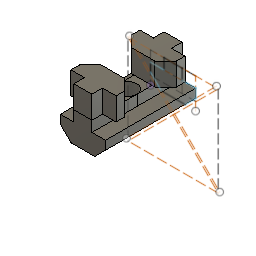
4040-t-conector v3 (Autodesk Fusion 360 design; units mm, degrees)
Autodesk Fusion 360 part; units mm, degrees
sketch "Sketch1" plane through (0, 0, 0) normal (0, 0, 1) x (1, 0, 0)
  line L0 (20, 0) -> (20, 13.5) construction
  line L1 (20, 13.5) -> (0, 13.5) construction
  line L2 (0, 13.5) -> (0, 0) construction
  line L3 (6, 13.5) -> (14, 13.5)
  line L4 (14, 13.5339) -> (14, 3.75) construction
  line L5 (14, 8.8) -> (6, 8.8) construction
  line L6 (6, 8.8) -> (6, 13.5) construction
  line L7 (0, 3.75) -> (20, 3.75) construction
  line L8 (-10, 13.5339) -> (30, 13.5339) construction
  line L9 (30, 13.5339) -> (30, -26.4661) construction
  line L10 (30, -26.4661) -> (-10, -26.4661) construction
  line L11 (-10, -26.4661) -> (-10, 13.5339) construction
  line L12 (-10, 13.5339) -> (30, -26.4661) construction
  line L13 (-9.2929, 14.241) -> (30.7071, -25.759) construction
  line L14 (30, 13.5339) -> (-10, -26.4661) construction
  line L15 (29.2929, 14.241) -> (-10.7071, -25.759) construction
  line L16 (0, 8.8) -> (20, 8.8) construction
  line L17 (6, 13.5) -> (6, 8.8)
  line L18 (0, 8.8) -> (0, 4.9481)
  line L19 (4.7481, 0.2) -> (15.2519, 0.2)
  line L20 (15.2519, 0.2) -> (20, 4.9481)
  line L21 (20, 4.9481) -> (20, 8.8)
  line L22 (20, 8.8) -> (14, 8.8)
  line L23 (14, 8.8) -> (14, 13.5)
  line L24 (6, 8.8) -> (0, 8.8)
  line L25 (0, 4.9481) -> (4.7481, 0.2)
  dimension "d1" = 20
  dimension "d2" = 13.5
  dimension "d3" = 8
  dimension "d4" = 4.7
  dimension "d5" = 6
  dimension "d6" = 9.75
  dimension "d7" = 40
  dimension "d8" = 40
  dimension "d9" = 10
  dimension "d10" = -1
  dimension "d11" = 1
  dimension "d21" = 13.3
  constraint vertical L0
  constraint horizontal L1
  constraint vertical L2
  constraint coincident L2.end origin
  constraint horizontal L3
  constraint vertical L4
  constraint horizontal L5
  constraint vertical L6
  constraint coincident L1 L3.start
  constraint coincident L2 L7.start
  constraint coincident L0 L7.end
  constraint perpendicular L0 L7
  constraint horizontal L8
  constraint vertical L9
  constraint horizontal L10
  constraint vertical L11
  constraint coincident L2 L16.start
  constraint coincident L0 L16.end
  constraint perpendicular L0 L16
  constraint coincident L13 L18.end
  constraint coincident L2 L18.end
  constraint coincident L13 L19.start
  constraint coincident L15 L19.end
  constraint coincident L15 L20.end
  constraint coincident L0 L20.end
  constraint coincident L7 L4.end
  constraint coincident L5.start L4
  constraint coincident L8 L4.start
  constraint coincident L3.end L4
  measures "d1" distance of L2.end L0.start
  measures "d2" distance of L2.end L1.end
  measures "d3" distance of L3.start L3.end
  measures "d4" distance of L3.start L5.end
  measures "d5" distance of L2 L6
  measures "d6" distance of L1 L7
  measures "d7" distance of L8.start L8.end
  measures "d8" distance of L8.start L10.end
  measures "d9" distance of L2 L11
  measures "d21" distance of L1 L19
extrude "Extrude1" add sketch "Sketch1" along normal blind 40 makes body 1
sketch "Sketch3" plane through (0, 0, 0) normal (0, 0, 1) x (1, 0, 0)
copy_body "CopyPasteBodies2" bodies 1 makes body 2
copy_body "CopyPasteBodies3" bodies 1 makes body 3
move_body "Move3" bodies 3 to x (1, 0, 0) y (0, 0, 1) z (0, -1, 0) at (0, 53.5, 26.5)
copy_body "CopyPasteBodies4" bodies 1 makes body 4
move_body "Move4" bodies 4 to x (1, 0, 0) y (0, 0, -1) z (0, 1, 0) at (0, 13.5, 13.5)
move_face "OffsetFaces1" offset -30 1 faces at (8.6667, 53.5, 29.5667) on bodies 3
move_face "OffsetFaces2" offset -20 1 faces at (8.6667, 53.5, 10.4333) on bodies 4
sketch "Sketch4" plane through (0, 13.5, 0) normal (0, 1, 0) x (-1, 0, 0)
  line L0 (-14, 0) -> (-6, 0)
  line L1 (-6, 0) -> (-6, 40)
  line L2 (-6, 40) -> (-14, 40)
  line L3 (-14, 40) -> (-14, 0)
  circle A0 centre (-10, 20) radius 4
  line L4 (0, 0) -> (0, 40)
  line L5 (-20, 0) -> (-20, 40)
  dimension "d16" = 8
  dimension "d17" = 20
  dimension "d18" = 10
  dimension "d22" = 20
  measures "d16" diameter of A0
  measures "d17" distance of L0 A0.centre
  measures "d18" distance of A0.centre L4
  measures "d22" distance of L4 L5
extrude "Extrude2" cut sketch "Sketch4" against normal blind 17 contours A0 bodies 1 2
combine "Combine1" operation add target body 3 tool bodies 1 4
copy_body "Body->Comp1" bodies 2 removing the originals makes body 5 in component "t-block"
move_face "OffsetFaces3" offset -10 1 faces at (8.6667, 33.5, 10.4333) on bodies 3
component "t-block" placed x (1, 0, 0) y (0, 1, 0) z (0, 0, 1) at (0, 0, 0)
equation "d5 = ( d1 - d3 ) / 2"
equation "d9 = ( d7 - d1 ) / 2"
equation "d18 = d22 / 2"
named bodies: "t-block"
